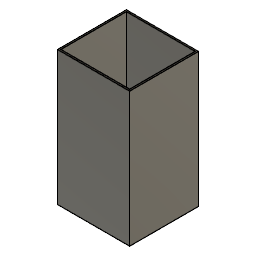
boitier_moteur_roue (Autodesk Fusion 360 design; units mm, degrees)
part number: 2026-05-21-08-46-45-224
Autodesk Fusion 360 part; units mm, degrees
note: some values were not read from the file. Set by a fixed rule: which sketch regions a step uses.
sketch "Esquisse1" plane through (0, 0, 0) normal (0, 0, 1) x (1, 0, 0)
  line L0 (0, 0) -> (22, 0)
  line L1 (22, 0) -> (22, 21)
  line L2 (22, 21) -> (0, 21)
  line L3 (0, 21) -> (0, 0)
  dimension "d1" = 22
  dimension "d2" = 21
  constraint horizontal L0
  constraint vertical L1
  constraint horizontal L2
  constraint vertical L3
  constraint coincident L0.start L3.end
  measures "d1" distance of L0.start L0.end
  measures "d2" distance of L0.start L2.end
extrude "Extrusion1" add sketch "Esquisse1" along normal blind 41
shell "Coque1" thickness 0.5 removed faces 1 at (7.3333, 7, 41)
sketch "Esquisse2" plane through (0, 0, 0) normal (0, 0, 1) x (1, 0, 0)
  line L0 (4.5, 20.5) -> (4.5, 15)
  line L1 (0, 15) -> (4.5, 15)
  circle A0 centre (4.5, 15) radius 2
  line L2 (22.5, 5) -> (18, 5)
  line L3 (18, -0.5) -> (18, 5)
  circle A1 centre (18, 5) radius 2
  dimension "d6" = 5.5
  dimension "d7" = 4.5
  dimension "d8" = 4
  dimension "d23" = 4.5
  dimension "d24" = 5.5
  dimension "d25" = 4
  constraint vertical L0
  constraint horizontal L1
  constraint coincident L0.end L1.end
  constraint horizontal L2
  constraint coincident L2.end L3.end
  constraint vertical L3
  measures "d6" distance of L0.start L0.end
  measures "d7" distance of L1.start L0.end
  measures "d8" diameter of A0
  measures "d23" distance of L2.start L2.end
  measures "d24" distance of L2.end L3.start
  measures "d25" diameter of A1
extrude "Extrusion2" cut sketch "Esquisse2" along normal blind 2
sketch "Esquisse3" plane through (0, 0, 0.5) normal (0, 0, 1) x (-1, 0, 0)
  circle A0 centre (-4.5, -15) radius 2
  line L0 (-0.5, -20.5) -> (-0.5, -0.5)
  line L1 (-0.5, -0.5) -> (-21.5, -0.5)
  line L2 (-21.5, -0.5) -> (-21.5, -20.5)
  line L3 (-21.5, -20.5) -> (-0.5, -20.5)
  line L4 (-11, -20.5) -> (-11, -11)
  circle A1 centre (-11, -11) radius 3.5
  circle A2 centre (-18, -5) radius 2
  dimension "d18" = 7
  constraint midpoint L3 L4.start
  constraint perpendicular L3 L4
  constraint coincident L4.end A1.centre
  measures "d18" diameter of A1
extrude "Extrusion3" cut sketch "Esquisse3" against normal blind 2 contours A1
